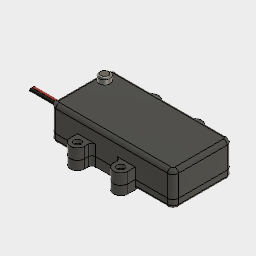
770 2xAA battery holder (Autodesk Fusion 360 design; units mm, degrees)
Autodesk Fusion 360 part; units mm, degrees
sketch "Sketch1" plane through (0, 0, 0) normal (0, 0, 1) x (1, 0, 0)
  line L0 (0, 0) -> (68, 0)
  line L1 (68, 0) -> (68, 33)
  line L2 (68, 33) -> (0, 33)
  line L3 (0, 33) -> (0, 0)
  dimension "d1" = 68
  dimension "d2" = 33
  measures "d1" distance of L0.start L0.end
  measures "d2" distance of L0.start L2.end
extrude "Extrude1" add sketch "Sketch1" along normal blind 19 makes body 1
fillet "Fillet1" radius 3 4 edges at (0, 0, 9.5) (68, 33, 9.5) (68, 0, 9.5) (0, 33, 9.5) on bodies 1
ref_plane "WorkPlane1" through (34, 16.5, 5) normal (0, 0, -1) x (-1, 0, 0)
split "Split1" by plane through (34, 16.5, 5) normal (0, 0, -1) bodies 1 makes body 2 at (44.3333, 11, 0)
ref_plane "WorkPlane2" through (34, 16.5, 11) normal (0, 0, 1) x (1, 0, 0)
ref_plane "WorkPlane3" through (34, 16.5, 12) normal (0, 1, 0) x (-1, 0, 0)
sketch "Sketch2" plane through (34, 16.5, 11) normal (0, 0, 1) x (1, 0, 0)
  arc A0 (-31, 16.5) -> (-34, 13.5) centre (-31, 13.5) ccw
  line L0 (-34, 13.5) -> (-34, -13.5)
  arc A1 (-34, -13.5) -> (-31, -16.5) centre (-31, -13.5) ccw
  line L1 (-31, -16.5) -> (31, -16.5)
  arc A2 (31, -16.5) -> (34, -13.5) centre (31, -13.5) ccw
  line L2 (34, -13.5) -> (34, 13.5)
  arc A3 (34, 13.5) -> (31, 16.5) centre (31, 13.5) ccw
  line L3 (31, 16.5) -> (-31, 16.5)
  line L4 (13, 24.5) -> (5, 24.5)
  line L5 (5, 24.5) -> (5, 16.5)
  line L6 (5, 16.5) -> (13, 16.5)
  line L7 (13, 16.5) -> (13, 24.5)
  line L8 (-11, 16.5) -> (-19, 16.5)
  line L9 (-19, 16.5) -> (-19, 24.5)
  line L10 (-19, 24.5) -> (-11, 24.5)
  line L11 (-11, 24.5) -> (-11, 16.5)
  circle A4 centre (9, 20.5) radius 2
  circle A5 centre (-15, 20.5) radius 2
  circle A6 centre (-15, 20.5) radius 1
  circle A7 centre (9, 20.5) radius 1
  dimension "d8" = 8
  dimension "d9" = 8
  dimension "d10" = 21
  dimension "d11" = 8
  dimension "d12" = 8
  dimension "d13" = 16
  dimension "d14" = 4
  dimension "d15" = 4
  dimension "d30" = 2
  dimension "d31" = 2
  measures "d8" distance of L4.start L4.end
  measures "d9" distance of L4.start L6.end
  measures "d10" distance of L2 L7
  measures "d11" distance of L8.start L8.end
  measures "d12" distance of L8.start L10.end
  measures "d13" distance of L5 L11
  measures "d14" diameter of A4
  measures "d15" diameter of A5
  measures "d30" diameter of A6
  measures "d31" diameter of A7
extrude "Extrude2" add sketch "Sketch2" against normal up to surface (6 mm away) contours L3 L8 L9 L10 L11 | L3 L4 L5 L6 L7 bodies 1
extrude "Extrude4" add sketch "Sketch2" along normal blind 4 from surface at -6 contours A4 | A5 bodies 1
mirror "Mirror1" about plane through (34, 16.5, 12) normal (0, 1, 0) of "Extrude2", "Extrude4"
fillet "Fillet2" radius 4 8 edges at (15, 41, 8) (23, 41, 8) (39, 41, 8) (47, 41, 8) (15, -8, 8) (23, -8, 8) (39, -8, 8) (47, -8, 8) on bodies 1
fillet "Fillet3" radius 2 4 edges at (39, 33, 8) (23, 33, 8) (23, 0, 8) (39, 0, 8) on bodies 1
sketch "Sketch3" plane through (0, 0, 0) normal (0, 0, -1) x (1, 0, 0)
  arc A0 (0, -30) -> (3, -33) centre (3, -30) ccw
  line L0 (3, -33) -> (65, -33)
  arc A1 (65, -33) -> (68, -30) centre (65, -30) ccw
  line L1 (68, -30) -> (68, -3)
  arc A2 (68, -3) -> (65, 0) centre (65, -3) ccw
  line L2 (65, 0) -> (3, 0)
  arc A3 (3, 0) -> (0, -3) centre (3, -3) ccw
  line L3 (0, -3) -> (0, -30)
  arc A4 (47, 4) -> (39, 4) centre (43, 4) ccw
  line L4 (39, 4) -> (39, 2)
  arc A5 (37, 0) -> (39, 2) centre (37, 2) ccw
  line L5 (37, 0) -> (25, 0)
  arc A6 (23, 2) -> (25, 0) centre (25, 2) ccw
  line L6 (23, 2) -> (23, 4)
  arc A7 (23, 4) -> (15, 4) centre (19, 4) ccw
  line L7 (15, 4) -> (15, 0)
  line L8 (15, 0) -> (3, 0)
  arc A8 (3, 0) -> (0, -3) centre (3, -3) ccw
  line L9 (0, -3) -> (0, -30)
  arc A9 (0, -30) -> (3, -33) centre (3, -30) ccw
  line L10 (3, -33) -> (15, -33)
  line L11 (15, -33) -> (15, -37)
  arc A10 (15, -37) -> (23, -37) centre (19, -37) ccw
  line L12 (23, -37) -> (23, -35)
  arc A11 (25, -33) -> (23, -35) centre (25, -35) ccw
  line L13 (25, -33) -> (37, -33)
  arc A12 (39, -35) -> (37, -33) centre (37, -35) ccw
  line L14 (39, -35) -> (39, -37)
  arc A13 (39, -37) -> (47, -37) centre (43, -37) ccw
  line L15 (47, -37) -> (47, -33)
  line L16 (47, -33) -> (65, -33)
  arc A14 (65, -33) -> (68, -30) centre (65, -30) ccw
  line L17 (68, -30) -> (68, -3)
  arc A15 (68, -3) -> (65, 0) centre (65, -3) ccw
  line L18 (65, 0) -> (47, 0)
  line L19 (47, 0) -> (47, 4)
  circle A16 centre (19, -37) radius 1
  circle A17 centre (43, -37) radius 1
  circle A18 centre (43, 4) radius 1
  circle A19 centre (19, 4) radius 1
  circle A20 centre (43, -37) radius 1
  circle A21 centre (19, -37) radius 1
  circle A22 centre (43, 4) radius 1
  circle A23 centre (19, 4) radius 1
  line L20 (43, 1) -> (45.5981, 2.5)
  line L21 (45.5981, 2.5) -> (45.5981, 5.5)
  line L22 (45.5981, 5.5) -> (43, 7)
  line L23 (43, 7) -> (40.4019, 5.5)
  line L24 (40.4019, 5.5) -> (40.4019, 2.5)
  line L25 (40.4019, 2.5) -> (43, 1)
  line L26 (43, -40) -> (45.5981, -38.5)
  line L27 (45.5981, -38.5) -> (45.5981, -35.5)
  line L28 (45.5981, -35.5) -> (43, -34)
  line L29 (43, -34) -> (40.4019, -35.5)
  line L30 (40.4019, -35.5) -> (40.4019, -38.5)
  line L31 (40.4019, -38.5) -> (43, -40)
  line L32 (19, -40) -> (21.5981, -38.5)
  line L33 (21.5981, -38.5) -> (21.5981, -35.5)
  line L34 (21.5981, -35.5) -> (19, -34)
  line L35 (19, -34) -> (16.4019, -35.5)
  line L36 (16.4019, -35.5) -> (16.4019, -38.5)
  line L37 (16.4019, -38.5) -> (19, -40)
  line L38 (19, 1) -> (21.5981, 2.5)
  line L39 (21.5981, 2.5) -> (21.5981, 5.5)
  line L40 (21.5981, 5.5) -> (19, 7)
  line L41 (19, 7) -> (16.4019, 5.5)
  line L42 (16.4019, 5.5) -> (16.4019, 2.5)
  line L43 (16.4019, 2.5) -> (19, 1)
  point P0 (43, 4)
  point P1 (43, -37)
  point P2 (19, -37)
  point P3 (19, 4)
  dimension "d24" = 2
  dimension "d25" = 2
  dimension "d26" = 2
  dimension "d27" = 2
  dimension "d35" = 3
  dimension "d36" = 3
  dimension "d37" = 3
  dimension "d38" = 3
  measures "d24" diameter of A16
  measures "d25" diameter of A17
  measures "d26" diameter of A18
  measures "d27" diameter of A19
  measures "d35" distance of L20.start P0
  measures "d36" distance of L26.start P1
  measures "d37" distance of L32.start P2
  measures "d38" distance of L38.start P3
extrude "Extrude3" add sketch "Sketch3" against normal up to surface (5 mm away) contours L0 L11 A10 L12 A11 | L2 A6 L6 A7 L7 | L0 A12 L14 A13 L15 | L2 A4 L4 A5 L19 | L20 L21 L22 L23 L24 L25 | L26 L27 L28 L29 L30 L31 | L32 L33 L34 L35 L36 L37 | L38 L39 L40 L41 L42 L43 bodies 2
extrude "Extrude5" cut sketch "Sketch3" against normal blind 3 contours L20 L21 L22 L23 L24 L25 | L26 L27 L28 L29 L30 L31 | L32 L33 L34 L35 L36 L37 | L38 L39 L40 L41 L42 L43 bodies 2
sketch "Sketch4" plane through (0, 0, 19) normal (0, 0, 1) x (-1, 0, 0)
  arc A0 (-3, -33) -> (0, -30) centre (-3, -30) ccw
  line L0 (0, -30) -> (0, -3)
  arc A1 (0, -3) -> (-3, 0) centre (-3, -3) ccw
  line L1 (-3, 0) -> (-65, 0)
  arc A2 (-65, 0) -> (-68, -3) centre (-65, -3) ccw
  line L2 (-68, -3) -> (-68, -30)
  arc A3 (-68, -30) -> (-65, -33) centre (-65, -30) ccw
  line L3 (-65, -33) -> (-3, -33)
  circle A4 centre (-5, -25) radius 3
  dimension "d42" = 6
  dimension "d43" = 5
  dimension "d44" = 8
  measures "d42" diameter of A4
  measures "d43" distance of L0 A4.centre
  measures "d44" distance of L3 A4.centre
extrude "Extrude6" add sketch "Sketch4" along normal blind 3.5 separate body contours A4 makes body 3
fillet "Fillet5" radius 1 1 edges at (7.797, 26.0848, 22.5) on bodies 3
sketch "Sketch5" plane through (0, 0, 0) normal (-1, 0, 0) x (0, -1, 0)
  line L0 (-30, 5) -> (-3, 5)
  line L1 (-3, 5) -> (-3, 19)
  line L2 (-3, 19) -> (-30, 19)
  line L3 (-30, 19) -> (-30, 5)
  circle A0 centre (-5, 15) radius 2.5
  arc A1 (-5, 14.5025) -> (-5, 15.4975) centre (-4.25, 15) ccw
  arc A2 (-5, 15.4975) -> (-5, 14.5025) centre (-5.75, 15) ccw
  line L4 (-5.75, 15) -> (-4.25, 15) construction
  dimension "d48" = 5
  dimension "d49" = 4
  dimension "d50" = 2
  dimension "d55" = 1.8
  dimension "d56" = 1.8
  dimension "d60" = 1.5
  measures "d48" diameter of A0
  measures "d49" distance of L2 A0.centre
  measures "d50" distance of L1 A0.centre
  measures "d55" diameter of A2
  measures "d56" diameter of A1
  measures "d60" distance of A2.centre A1.centre
extrude "Extrude7" cut sketch "Sketch5" against normal blind 1 contours L1 A0 | L1 A0 | A1 A2 bodies 1
extrude "Extrude8" add sketch "Sketch5" along normal blind 16 from surface at -1 contours A1 A2 bodies 1
fillet "Fillet4" radius 2 18 edges at (0.8787, 0.8787, 19) (34, 0, 19) (67.1213, 0.8787, 19) (68, 16.5, 19) (67.1213, 32.1213, 19) (34, 33, 19) (0.8787, 32.1213, 19) (0, 16.5, 19) (9, 33, 0) (0.8787, 32.1213, 0) (0, 16.5, 0) (0.8787, 0.8787, 0) (9, 0, 0) (56, 0, 0) (67.1213, 0.8787, 0) (68, 16.5, 0) (67.1213, 32.1213, 0) (56, 33, 0) on bodies 1 2
